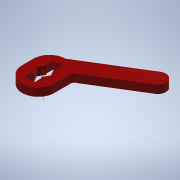
# Autodesk Inventor part: В. шарн. - держатель соединителя
Saved by Autodesk Inventor 2020 (Build 240168000, 168)
## iProperties
Created: 2020-02-23
Part Number: В. шарн. - держатель соединителя
Material: Типовые
Document SubType Name: Modeling
Designer: Leancher
Density: 1 g/cm^3
Appearance: По умолчанию
Author: Leancher
Autodesk Inventor part; units mm, degrees
ref_plane "YZ Plane" through (0, 0, 0) normal (1, 0, 0) x (0, 1, 0)
ref_plane "XZ Plane" through (0, 0, 0) normal (0, 1, 0) x (-1, 0, 0)
ref_plane "XY Plane" through (0, 0, 0) normal (0, 0, 1) x (1, 0, 0)
sketch "Эскиз1" plane through (0, 0, 0) normal (0, 0, 1) x (1, 0, 0)
  arc A0 (5.088, 16.8311) -> (-4.912, 6.8311) centre (5.088, 6.8311) ccw
  line L0 (7.3397, 7.2282) -> (8.088, 7.2282)
  line L1 (7.3397, 7.2282) -> (9.538, 3.3282)
  line L2 (2.8364, 7.2282) -> (0.638, 3.3282)
  line L3 (7.3397, -0.5718) -> (9.538, 3.3282)
  line L4 (2.8364, -0.5718) -> (0.638, 3.3282)
  line L5 (2.088, 12.1282) -> (8.088, 12.1282)
  line L6 (8.088, 12.1282) -> (8.088, 7.2282)
  line L7 (2.088, 7.2282) -> (2.8364, 7.2282)
  line L8 (2.088, 12.1282) -> (2.088, 7.2282)
  line L9 (-4.912, 6.8311) -> (-4.912, -0.1747)
  arc A1 (-4.912, -0.1747) -> (15.088, -0.1747) centre (5.088, -0.1747) ccw
  line L10 (15.088, -0.1747) -> (15.088, 10.1176)
  line L11 (7.3397, -0.5718) -> (8.088, -0.5718)
  line L12 (2.088, -5.4718) -> (8.088, -5.4718)
  line L13 (8.088, -5.4718) -> (8.088, -0.5718)
  line L14 (2.088, -0.5718) -> (2.8364, -0.5718)
  line L15 (2.088, -5.4718) -> (2.088, -0.5718)
  line L16 (5.088, 16.8311) -> (41.732, 39.3305)
  line L17 (46.9644, 30.8087) -> (16.0416, 11.822)
  arc A2 (48.6091, 37.6858) -> (41.732, 39.3305) centre (44.3482, 35.0696) ccw
  arc A3 (46.9644, 30.8087) -> (48.6091, 37.6858) centre (44.3482, 35.0696) ccw
  arc A4 (16.0416, 11.822) -> (15.088, 10.1176) centre (17.088, 10.1176) ccw
  point P0 (5.088, 3.3282)
  point P1 (15.088, 11.2365)
  constraints: 38 end point, 10 point on circle, 5 centre point, 2 point on line, 2 tangent, 1 vertical
extrude "Выдавливание1" add sketch "Эскиз1" along normal blind 5
